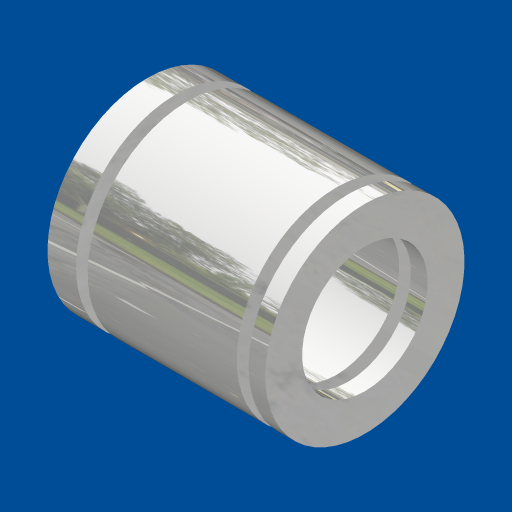
# Autodesk Inventor part: baseSpacers
Saved by Autodesk Inventor 2023 (Build 270158030, 158C)
## iProperties
Created: 2023-03-03
Part Number: baseSpacers
Material: Aluminum 6061
Document SubType Name: Modeling
Designer: kumpu
Density: 2.7 g/cm^3
Appearance: Aluminum - Dark
Author: kumpu
Autodesk Inventor part; units mm, degrees
ref_plane "YZ Plane" through (0, 0, 0) normal (1, 0, 0) x (0, 1, 0)
ref_plane "XZ Plane" through (0, 0, 0) normal (0, 1, 0) x (-1, 0, 0)
ref_plane "XY Plane" through (0, 0, 0) normal (0, 0, 1) x (1, 0, 0)
sketch "Sketch1" plane through (0, 0, 0) normal (0, 0, 1) x (1, 0, 0)
  line L0 (-29.25, 25.4) -> (-22, 25.4)
  line L1 (-22, 25.4) -> (-22, 16)
  line L2 (-22, 16) -> (-29.25, 16)
  line L3 (-29.25, 16) -> (-29.25, 25.4)
  line L4 (-19, 25.4) -> (19, 25.4)
  line L5 (19, 25.4) -> (19, 16)
  line L6 (19, 16) -> (-19, 16)
  line L7 (-19, 16) -> (-19, 25.4)
  line L8 (22, 25.4) -> (26.25, 25.4)
  line L9 (26.25, 25.4) -> (26.25, 16)
  line L10 (26.25, 16) -> (22, 16)
  line L11 (22, 16) -> (22, 25.4)
  line L12 (-29.25, 0) -> (26.25, 0)
  line L13 (0, 16) -> (0, 0) construction
  dimension "d0" = 3
  dimension "d1" = 3
  dimension "d2" = 38
  dimension "d3" = 7.25
  dimension "d4" = 50.8
  dimension "d5" = 32
  dimension "d6" = 26.25
  constraints: 28 end point, 6 parallel, 4 horizontal, 4 point on line, 3 collinear, 3 perpendicular, 1 midpoint, 1 vertical
  measures "d0" distance between parallel lines of L1 L7
  measures "d1" distance between parallel lines of L5 L11
  measures "d2" distance of L4.start L4.end
  measures "d3" distance of L0.start L0.end
  measures "d4" diameter of L0 L12
  measures "d5" diameter of L2 L12
  measures "d6" distance between parallel lines of L9 L13
revolve "Revolution1" add sketch "Sketch1" angle 360 about axis through (-29.25, 0, 0) along (1, 0, 0)
equation "\"d1\" = d0"
body "Solid1"
